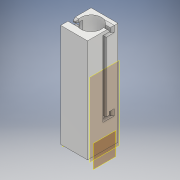
# Autodesk Inventor part: RescueKitThrow_pipe
Saved by Autodesk Inventor 2018.3 (Build 223284000, 284)
## iProperties
Created: 2019-02-10
Part Number: RescueKitThrow_pipe
Material: ABS プラスチック
Document SubType Name: Modeling
Designer: shun2
Density: 1.06 g/cm^3
Appearance: 滑らか - 白
Author: shun2
Autodesk Inventor part; units mm, degrees
ref_plane "YZ Plane" through (0, 0, 0) normal (1, 0, 0) x (0, 1, 0)
ref_plane "XZ Plane" through (0, 0, 0) normal (0, 1, 0) x (-1, 0, 0)
ref_plane "XY Plane" through (0, 0, 0) normal (0, 0, 1) x (1, 0, 0)
sketch "スケッチ1" plane through (0, 0, 0) normal (0, 0, 1) x (1, 0, 0)
  circle A0 centre (0, 0) radius 0.6
  line L0 (-0.6, 0) -> (0.6, 0)
  line L1 (-0.6, 0) -> (0.6, 0)
  line L2 (-13, 13) -> (13, 13)
  line L3 (13, 13) -> (13, -13)
  line L4 (13, -13) -> (-13, -13)
  line L5 (-13, -13) -> (-13, 13)
  dimension "d1" = 1.2
  dimension "d57" = 26
  dimension "d58" = 26
  constraints: 12 end point, 3 horizontal, 2 parallel, 2 point on circle, 1 centre point, 1 perpendicular
  measures "d1" diameter of A0
  measures "d57" distance of L3.end L4.end
  measures "d58" distance of L2.end L3.end
extrude "押し出し1" add sketch "スケッチ1" along normal blind 20 contours L0 A0 | L2 L3 L4 L5 picked at (0.1497, 0.1326)
sketch "スケッチ2" plane through (0, 0, 20) normal (0, 0, 1) x (1, 0, 0)
  circle A0 centre (0, 0) radius 0.6 projected
  circle A1 centre (0, 0) radius 10
  line L0 (-0.6, 0) -> (0.6, 0)
  line L1 (13, 0) -> (13, 13)
  line L2 (-0.6, 0) -> (0.6, 0)
  line L3 (-13, 13) -> (13, 13)
  line L4 (13, 13) -> (13, -13)
  line L5 (13, -13) -> (-13, -13)
  line L6 (-13, -13) -> (-13, 13)
  dimension "d5" = 20
  dimension "d59" = 26
  dimension "d60" = 26
  constraints: 14 end point, 3 horizontal, 2 parallel, 2 perpendicular, 2 point on circle, 1 centre point, 1 coincident
  measures "d5" diameter of A1
  measures "d59" distance of L4.end L5.end
  measures "d60" distance of L3.end L4.end
extrude "押し出し2" add sketch "スケッチ2" along normal blind 80 contours L4 L5 L6 L3 L1
ref_plane "作業平面3" through (13, -13, 0) normal (1, 0, 0) x (0, 0, -1)
ref_plane "作業平面4" through (13, 0, 0) normal (1, 0, 0) x (0, 1, 0)
sketch "スケッチ3" plane through (13, 0, 0) normal (1, 0, 0) x (0, 1, 0)
  line L0 (-13, 0) -> (13, 0) projected
  line L1 (-13, 0) -> (-13, 65) projected
  line L2 (1.5, 94) -> (-1.5, 94)
  line L3 (-1.5, 94) -> (-1.5, 24)
  line L4 (-1.5, 24) -> (1.5, 24)
  line L5 (1.5, 24) -> (1.5, 94)
  line L6 (-13, 100) -> (13, 100) projected
  point P0 (0, 0)
  point P1 (0, 0)
  point P2 (0, 0)
  dimension "d80" = 3
  dimension "d81" = 70
  dimension "d90" = 6
  constraints: 8 end point, 2 parallel, 1 horizontal, 1 perpendicular, 1 other
  measures "d80" distance of L4.end L3.end
  measures "d81" distance of L3.end L2.end
  measures "d90" distance between parallel lines of L2 L6
extrude "押し出し3" cut sketch "スケッチ3" against normal blind 30
ref_plane "作業平面5" through (13, 0, 0) normal (1, 0, 0) x (0, 1, 0)
sketch "スケッチ4" plane through (13, 0, 0) normal (1, 0, 0) x (0, 1, 0)
  line L0 (-1.5, 94) -> (1.5, 94) projected
  line L1 (-1.5, 94) -> (7.5, 94)
  line L2 (7.5, 94) -> (7.5, 97)
  line L3 (4.5, 97) -> (-1.5, 97)
  line L4 (-1.5, 97) -> (-1.5, 94)
  line L5 (7.5, 94) -> (4.5, 94)
  line L6 (4.5, 97) -> (4.5, 100)
  line L7 (4.5, 100) -> (7.5, 100)
  line L8 (7.5, 100) -> (7.5, 94)
  line L9 (-1.5, 24) -> (-1.5, 94) projected
  line L10 (-1.5, 24) -> (7.5, 24)
  line L11 (7.5, 24) -> (7.5, 27)
  line L12 (4.5, 27) -> (-1.5, 27)
  line L13 (-1.5, 27) -> (-1.5, 24)
  line L14 (7.5, 24) -> (4.5, 24)
  line L15 (4.5, 27) -> (4.5, 30)
  line L16 (4.5, 30) -> (7.5, 30)
  line L17 (7.5, 30) -> (7.5, 24)
  point P0 (0, 0)
  point P1 (-1.25, 59)
  point P2 (-1.25, 10)
  dimension "d82" = 9
  dimension "d83" = 3
  dimension "d84" = 3
  dimension "d85" = 6
  dimension "d86" = 9
  dimension "d87" = 3
  dimension "d88" = 3
  dimension "d89" = 6
  constraints: 32 end point, 8 parallel, 4 horizontal, 4 perpendicular
  measures "d82" distance of L3.end L2.end
  measures "d83" distance of L2.end L1.end
  measures "d84" distance of L6.end L7.end
  measures "d85" distance of L5.end L6.end
  measures "d86" distance of L12.end L11.end
  measures "d87" distance of L11.end L10.end
  measures "d88" distance of L15.end L16.end
  measures "d89" distance of L14.end L15.end
extrude "押し出し4" cut sketch "スケッチ4" against normal blind 8
ref_plane "作業平面2" through (-13, 0, 0) normal (1, 0, 0) x (0, 1, 0)
sketch "スケッチ5" plane through (-13, 0, 0) normal (1, 0, 0) x (0, 1, 0)
  line L0 (6.25, 10) -> (-1.25, 10) projected
  line L1 (1.5, 94) -> (1.5, 27) projected
  line L2 (1.5, 94) -> (-7.5, 94)
  line L3 (-7.5, 94) -> (-7.5, 97)
  line L4 (-4.5, 97) -> (1.5, 97)
  line L5 (1.5, 97) -> (1.5, 94)
  line L6 (-7.5, 94) -> (-4.5, 94)
  line L7 (-4.5, 97) -> (-4.5, 100)
  line L8 (-4.5, 100) -> (-7.5, 100)
  line L9 (-7.5, 100) -> (-7.5, 94)
  line L10 (-1.5, 24) -> (1.5, 24) projected
  line L11 (1.5, 24) -> (-7.5, 24)
  line L12 (-7.5, 24) -> (-7.5, 27)
  line L13 (-4.5, 27) -> (1.5, 27)
  line L14 (1.5, 27) -> (1.5, 24)
  line L15 (-7.5, 24) -> (-4.5, 24)
  line L16 (-4.5, 27) -> (-4.5, 30)
  line L17 (-4.5, 30) -> (-7.5, 30)
  line L18 (-7.5, 30) -> (-7.5, 24)
  point P0 (0, 0)
  point P1 (1.25, 10)
  dimension "d91" = 9
  dimension "d92" = 3
  dimension "d93" = 3
  dimension "d94" = 6
  dimension "d95" = 9
  dimension "d96" = 3
  dimension "d97" = 3
  dimension "d98" = 6
  constraints: 32 end point, 8 parallel, 4 horizontal, 4 perpendicular, 1 point on line
  measures "d91" distance of L3.end L4.end
  measures "d92" distance of L2.end L3.end
  measures "d93" distance of L8.end L7.end
  measures "d94" distance of L7.end L6.end
  measures "d95" distance of L12.end L13.end
  measures "d96" distance of L11.end L12.end
  measures "d97" distance of L17.end L16.end
  measures "d98" distance of L16.end L15.end
extrude "押し出し5" cut sketch "スケッチ5" along normal blind 8
chamfer "面取り2" distance 2 angle 45 4 edges at (9.8072, 7.5, 100) (10.9651, 4.5, 100) (-10.9651, -4.5, 100) (-9.8072, -7.5, 100)
chamfer "面取り3" distance 2 angle 45 8 edges at (-13, -7.5, 96) (8.9303, 4.5, 97.5) (13, 7.5, 96) (-8.9303, -4.5, 97.5) (-13, -7.5, 27) (8.9303, 4.5, 28.5) (-8.9303, -4.5, 28.5) (13, 7.5, 27)
sketch "スケッチ6" plane through (0, 0, 20) normal (0, 0, 1) x (1, 0, 0)
  circle A0 centre (0, 0) radius 4.75
  dimension "d65" = 9.5
  constraints: 1 centre point, 1 coincident
  measures "d65" diameter of A0
extrude "押し出し6" cut sketch "スケッチ6" against normal blind 15
sketch "スケッチ7" plane through (-13, -13, 0) normal (0, -1, 0) x (1, 0, 0)
  line L0 (26, 0) -> (0, 0) projected
  line L1 (26, 0) -> (26, 100) projected
  line L2 (0, 100) -> (26, 100) projected
  line L3 (0, 0) -> (0, 100) projected
  point P0 (13, 0)
extrude "押し出し7" add sketch "スケッチ7" along normal blind 3.5
